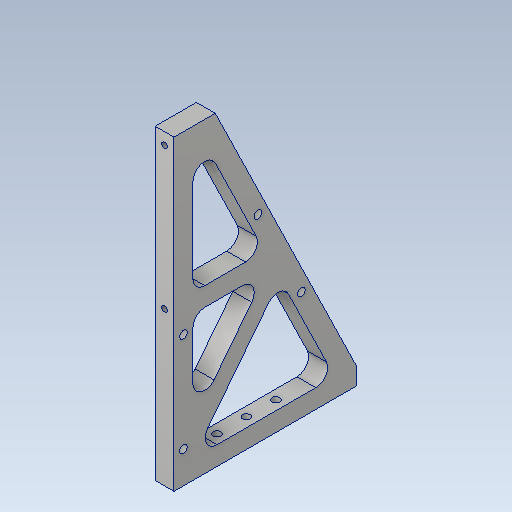
# Autodesk Inventor part: FAB-P0042 - Camera Bracket sCMOS
Saved by Autodesk Inventor 2020 (Build 240168000, 168)
## iProperties
Created: 2012-07-23
Part Number: FAB-P0042 - Camera Bracket sCMOS
Material: Aluminum 6061
Document SubType Name: Modeling
Designer: map
Density: 2.7 g/cm^3
Appearance: Aluminum - Flat
Mass: 606.914 g
Surface Area: 550.767 cm^2
Volume: 224.783 cm^3
Sending System: SolidWorks 2015
Last Author: ml2377
Last Saved: 2016-03-24
thickness: 16.000 mm
Author: map
Autodesk Inventor part; units mm, degrees
ref_plane "YZ Plane" through (0, 0, 0) normal (1, 0, 0) x (0, 1, 0)
ref_plane "XZ Plane" through (0, 0, 0) normal (0, 1, 0) x (-1, 0, 0)
ref_plane "XY Plane" through (0, 0, 0) normal (0, 0, 1) x (1, 0, 0)
derived "__05_Detection_MASTER__.ipt"
sketch "Sketch1_1" plane through (0, 0, 0) normal (0, 0, 1) x (1, 0, 0)
  line L0 (-119.8204, -325) -> (119.8204, -325)
  line L1 (0, 0) -> (0, -325) construction
  line L2 (-50, -75) -> (50, -75)
  line L3 (50, -75) -> (50, -195)
  line L4 (50, -195) -> (-50, -195)
  line L5 (-50, -195) -> (-50, -75)
  line L6 (-22.9, -88) -> (114.26, -88)
  line L7 (-37.5, -94.5) -> (37.5, -94.5)
  line L8 (-40.82, -88) -> (132.18, -88) construction
  point P0 (0, -75)
  point P1 (0, -94.5)
  point P2 (0, -94.5)
  point P3 (45.68, -88)
sketch "Sketch1" plane through (0, 0, 0) normal (1, 0, 0) x (0, 1, 0)
  line L0 (-325, 0) -> (-325, -155)
  line L1 (-325, 0) -> (-65, 0)
  line L2 (-311.0365, -155) -> (-65, -35)
  line L3 (-203, -16) -> (-309, -16)
  line L4 (-309, -16) -> (-309, -136.2051)
  line L5 (-309, -136.2051) -> (-214.2771, -90.0057)
  line L6 (-203, -16) -> (-203, -78.512)
  line L7 (-65, 0) -> (-65, -35)
  line L8 (-311.0365, -155) -> (-325, -155)
  line L9 (-187, -16) -> (-81, -16)
  line L10 (-81, -16) -> (-81, -25.0021)
  line L11 (-81, -25.0021) -> (-187, -76.7017)
  line L12 (-187, -76.7017) -> (-187, -16)
  line L13 (-195, 0) -> (-195, -109.6814) construction
  line L14 (-283.0117, -16) -> (-203, -78.512)
  line L15 (-309, -16) -> (-214.2771, -90.0057)
  line L16 (-296.0058, -16) -> (-195, -94.9144) construction
  dimension "d56" = 26
  dimension "d57" = 16
  dimension "d59" = 16
  dimension "d60" = 16
  dimension "d62" = 260
  dimension "d67" = 16
  dimension "d71" = 106
  dimension "d88" = 155
  dimension "d89" = 35
  dimension "d90" = 16
  dimension "d97" = 16
  dimension "d100" = 52
  constraints: 34 end point, 4 vertical, 3 point on line, 2 collinear, 2 horizontal, 2 parallel, 2 perpendicular, 1 coincident, 2 other
  measures "d56" angle of L2 L1
  measures "d57" distance between parallel lines of L1 L3
  measures "d59" distance between parallel lines of L0 L4
  measures "d60" distance between parallel lines of L2 L5
  measures "d62" distance between parallel lines of L0 L7
  measures "d67" distance between parallel lines of L12 L6
  measures "d71" distance between parallel lines of L4 L6
  measures "d88" distance of L0.start L0.end
  measures "d89" distance of L1.end L2.end
  measures "d90" distance between parallel lines of L7 L10
  measures "d97" distance between parallel lines of L14 L15
  measures "d100" angle of L14 L6
extrude "Extrusion1" add sketch "Sketch1" along normal mid plane 16
sketch "Sketch2" plane through (-8, -309, -136.2051) normal (0, 1, 0) x (1, 0, 0)
  line L0 (8, -91.8061) -> (8, -41.8061)
  point P0 (8, -66.8061)
  point P1 (8, -136.2051)
  dimension "d47" = 50
  dimension "d61" = 44.399
  constraints: 2 end point, 1 midpoint, 1 point on line, 1 vertical
  measures "d47" distance of L0.start L0.end
  measures "d61" distance of L0.start point (8, -136.205)
hole "M6Clearance" at (0, -309, -44.399) at (0, -309, -69.399) at (0, -309, -94.399) direction (0, -1, 0) diameter 6.6 end through all clearance for "Socket Head Cap Screw ISO 4762" size "M6" standard "ISO"
sketch "Sketch5" plane through (-8, -325, 0) normal (0, 0, 1) x (1, 0, 0)
  line L0 (8, 325) -> (8, 0) construction
  line L1 (-42, 250) -> (58, 250) projected
  line L2 (58, 130) -> (-42, 130) projected
  point P0 (8, 250)
  point P1 (8, 130)
  point P2 (8, 144.8749)
  point P3 (8, 250)
  point P4 (8, 130)
  constraints: 2 coincident, 2 midpoint, 2 point on line
hole "M6Tapped" at (0, -195, 0) at (0, -75, 0) direction (0, 0, -1) diameter 4.917 depth 17.1 tip angle 118 thread size "M6x1" class "6H" standard "ISO Metric profile"
fillet "Fillet7" radius 10 10 edges at (0, -203, -16) (0, -203, -78.512) (0, -309, -136.2051) (0, -187, -16) (0, -187, -76.7017) (0, -81, -16) (0, -81, -25.0021) (0, -283.0117, -16) (0, -214.2771, -90.0057) (0, -309, -16)
sketch "Sketch9" plane through (8, 0, 0) normal (1, 0, 0) x (0, 0, -1)
  line L0 (71.0928, -157.2507) -> (107.916, -232.7493)
  line L1 (155, -311.0365) -> (35, -65) construction
  line L2 (34.9879, -101.474) -> (69.6863, -172.6163) construction
  line L3 (97.0211, -228.6608) -> (129.1897, -294.6163) construction
  line L4 (60.6984, -187) -> (26, -187) construction
  line L5 (26, -203) -> (58.0089, -203) construction
  line L6 (56.4182, -145.4125) -> (70.7989, -138.3986) construction
  line L7 (0, -325) -> (155, -325) projected
  line L8 (16, -253.9696) -> (16, -213) construction
  line L9 (0, -65) -> (0, -325) construction
  line L10 (0, -228.2708) -> (16, -228.2708) construction
  line L11 (16, -213) -> (16, -253.9696) construction
  line L12 (8, -214) -> (8, -298)
  line L13 (120.2018, -309) -> (36.503, -309) projected
  point P0 (0, 0)
  point P1 (86.9541, -208.0204)
  point P2 (63.6085, -141.9055)
  point P3 (8, -228.2708)
  point P4 (8, -256)
  point P5 (89.7465, -213.7457)
  point P6 (16, -287.4345)
  point P7 (19.4554, -309)
  point P8 (100.103, -234.9796)
  point P9 (45.0842, -309)
  point P10 (16, -309)
  dimension "d72" = 84
  dimension "d83" = 84
  dimension "d93" = 29.7493
  dimension "d94" = 29.7493
  dimension "d98" = 53
  dimension "d99" = 53
  constraints: 8 end point, 6 point on line, 3 midpoint, 2 parallel, 1 horizontal, 1 perpendicular, 1 vertical
  measures "d72" distance of L0.start L0.end
  measures "d83" distance of L12.start L12.end
  measures "d93" distance from line of L0.end L5
  measures "d94" distance from line of L0.start L4
  measures "d98" distance from line of L5 point (8, -256)
  measures "d99" distance from line of L13 point (8, -256)
hole "Hole8" at (8, -157.2507, -71.0928) at (8, -232.7493, -107.916) at (8, -214, -8) at (8, -298, -8) direction (-1, 0, 0) diameter 6.6 end through all clearance for "Socket Head Cap Screw ISO 4762" size "M6" standard "ISO"
equation "\"d59\" = d57"
equation "\"d60\" = d57"
equation "\"d67\" = d57"
equation "\"d90\" = d57"
equation "\"d97\" = d57"
equation "\"d83\" = d72"
equation "\"d93\" = d94"
equation "\"d98\" = d99"
equation "\"d96\" = d57"
body "Solid3"
